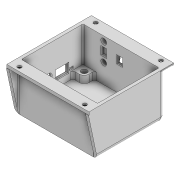
# Autodesk Inventor part: Temp
Saved by Autodesk Inventor 2021.2 (Build 252289000, 289)
## iProperties
Created: 2023-12-02
Part Number: Temp
Material: Типовые
Document SubType Name: Modeling
Designer: Egor
Density: 1 g/cm^3
Appearance: По умолчанию
Author: Egor
Autodesk Inventor part; units mm, degrees
ref_plane "YZ Plane" through (0, 0, 0) normal (1, 0, 0) x (0, 1, 0)
ref_plane "XZ Plane" through (0, 0, 0) normal (0, 1, 0) x (-1, 0, 0)
ref_plane "XY Plane" through (0, 0, 0) normal (0, 0, 1) x (1, 0, 0)
sketch "Эскиз1" plane through (0, 0, 0) normal (0, 1, 0) x (-1, 0, 0)
  line L0 (0, -50) -> (58, -50)
  line L1 (-2, -2) -> (-2, -48)
  line L2 (58, 0) -> (0, 0)
  line L3 (60, -48) -> (60, -2)
  line L4 (-2, 0) -> (60, 0)
  line L5 (60, 0) -> (60, -50)
  line L6 (60, -50) -> (-2, -50)
  line L7 (-2, -50) -> (-2, 0)
  circle A0 centre (2, -4) radius 1.6
  circle A1 centre (55, -4) radius 1.6
  circle A2 centre (55, -46) radius 1.6
  circle A3 centre (2, -46) radius 1.6
  circle A4 centre (2, -4) radius 1.6
  circle A5 centre (55, -4) radius 1.6
  circle A6 centre (55, -46) radius 1.6
  circle A7 centre (2, -46) radius 1.6
  circle A8 centre (2, -4) radius 2.4
  circle A9 centre (2, -4) radius 4
  circle A10 centre (55, -4) radius 4
  circle A11 centre (55, -4) radius 2.4
  circle A12 centre (55, -46) radius 4
  circle A13 centre (55, -46) radius 2.4
  circle A14 centre (2, -46) radius 4
  circle A15 centre (2, -46) radius 2.4
  dimension "d0" = 4.8
  dimension "d1" = 8
  dimension "d2" = 4.8
  dimension "d3" = 8
  dimension "d4" = 4.8
  dimension "d5" = 8
  dimension "d6" = 4.8
  dimension "d7" = 8
  constraints: 16 centre point, 16 end point, 9 coincident, 4 concentric, 2 parallel, 1 horizontal, 1 perpendicular, 1 point on line
  measures "d0" diameter of A8
  measures "d1" diameter of A9
  measures "d2" diameter of A11
  measures "d3" diameter of A10
  measures "d4" diameter of A13
  measures "d5" diameter of A12
  measures "d6" diameter of A15
  measures "d7" diameter of A14
extrude "Выдавливание1" add sketch "Эскиз1" along normal blind 2.5 contours L6 L7 L1 A14 L0 | A12 | A10 | A14 L1 A9 L2 L4 L5 L3 L6 L0 | A14 | L1 L7 L4 L2 A9 | A9 | A0 | A1 | A2 | A3 | A8 | A11 | A13 | A15
extrude "Выдавливание2" add sketch "Эскиз1" along normal blind 8.5 contours A12 | A10 | A14 | A9
sketch "Эскиз2" plane through (0, 0, 0) normal (0, -1, 0) x (1, 0, 0)
  line L0 (-60, 0) -> (2, 0) projected
  line L1 (2, 0) -> (2, -50) projected
  line L2 (2, -50) -> (-60, -50) projected
  line L3 (-60, -50) -> (-60, 0) projected
  line L4 (2, 0) -> (2, -50) projected
  line L5 (2.5, -50.5) -> (-60.5, -50.5)
  line L6 (-60.5, -50.5) -> (-60.5, 0.5)
  line L7 (-60.5, 0.5) -> (2.5, 0.5)
  line L8 (2.5, 0.5) -> (2.5, -50.5)
  line L9 (5, -50.5) -> (5, -53)
  line L10 (5, -53) -> (2.5, -53)
  line L11 (5, -53) -> (-63, -53)
  line L12 (-63, -53) -> (-63, 3)
  line L13 (-63, 3) -> (5, 3)
  line L14 (5, 3) -> (5, -53)
  point P0 (0, 0)
  dimension "d14" = 63
  dimension "d15" = 51
  dimension "d16" = 2.5
  dimension "d17" = 2.5
  dimension "d18" = 68
  dimension "d19" = 56
  constraints: 20 end point, 4 parallel, 2 horizontal, 2 perpendicular
  measures "d14" distance of L6.end L7.end
  measures "d15" distance of L5.end L6.end
  measures "d16" distance of L9.end L10.end
  measures "d17" distance of L9.start L9.end
  measures "d18" distance of L12.end L13.end
  measures "d19" distance of L11.end L12.end
extrude "Выдавливание3" add sketch "Эскиз2" against normal blind 2.5 contours L5 L6 L7 L8
extrude "Выдавливание4" add sketch "Эскиз2" against normal blind 35 contours L9 L10 L11 L12 L13 L14
sketch "Эскиз3" plane through (-63, 0, 3) normal (0, 0, 1) x (1, 0, 0)
  line L0 (0, 0) -> (0, 35) projected
  line L1 (0, 35) -> (68, 35)
  line L2 (68, 35) -> (68, 50)
  line L3 (68, 50) -> (0, 50)
  line L4 (0, 50) -> (0, 35)
  point P0 (63, 0)
  dimension "d24" = 15
  constraints: 8 end point, 2 parallel, 1 horizontal, 1 perpendicular
  measures "d24" distance of L2.end L1.end
extrude "Выдавливание5" add sketch "Эскиз3" against normal blind 150
sketch "Эскиз4" plane through (-63, 50, 3) normal (0, 1, 0) x (1, 0, 0)
  line L0 (0, 0) -> (0, 56) projected
  line L1 (68, 0) -> (68, 150) projected
  line L2 (0, 0) -> (68, 0)
  line L3 (68, 0) -> (68, 150)
  line L4 (68, 150) -> (0, 150)
  line L5 (0, 150) -> (0, 0)
  point P0 (63, 3)
  constraints: 8 end point, 2 parallel, 1 horizontal, 1 perpendicular
extrude "Выдавливание6" cut sketch "Эскиз4" against normal blind 2.5
sketch "Эскиз5" plane through (-63, 47.5, 3) normal (0, 1, 0) x (1, 0, 0)
  line L0 (0, 56) -> (0, 150) projected
  line L1 (0, 150) -> (10, 150)
  line L2 (10, 150) -> (10, 140)
  line L3 (10, 140) -> (0, 140)
  line L4 (0, 140) -> (0, 150)
  line L5 (68, 150) -> (0, 150) projected
  line L6 (68, 150) -> (58, 150)
  line L7 (58, 150) -> (58, 140)
  line L8 (58, 140) -> (68, 140)
  line L9 (68, 140) -> (68, 150)
  line L10 (0, 0) -> (0, 56) projected
  line L11 (0, 0) -> (10, 0)
  line L12 (10, 0) -> (10, 10)
  line L13 (10, 10) -> (0, 10)
  line L14 (0, 10) -> (0, 0)
  line L15 (10, 10) -> (58, 10)
  line L16 (58, 10) -> (58, 140)
  line L17 (58, 140) -> (10, 140)
  line L18 (10, 140) -> (10, 10)
  point P0 (63, 3)
  dimension "d29" = 10
  dimension "d30" = 10
  dimension "d31" = 10
  dimension "d32" = 10
  dimension "d33" = 10
  dimension "d34" = 10
  constraints: 32 end point, 8 parallel, 4 horizontal, 4 perpendicular
  measures "d29" distance of L2.end L3.end
  measures "d30" distance of L1.end L2.end
  measures "d31" distance of L8.end L7.end
  measures "d32" distance of L7.end L6.end
  measures "d33" distance of L13.end L12.end
  measures "d34" distance of L12.end L11.end
extrude "Выдавливание7" cut sketch "Эскиз5" against normal blind 10 contours L17 L16 L15 L18
sketch "Эскиз6" plane through (-63, 37.5, 3) normal (0, 1, 0) x (1, 0, 0)
  line L0 (58, 140) -> (10, 140) projected
  line L1 (10, 140) -> (10, 10) projected
  line L2 (10, 10) -> (58, 10) projected
  line L3 (58, 10) -> (58, 140) projected
  line L4 (0, 150) -> (68, 150) projected
  line L5 (68, 150) -> (68, 0) projected
  line L6 (68, 0) -> (0, 0) projected
  line L7 (0, 0) -> (0, 150) projected
  line L8 (68, 56) -> (0, 56) projected
  line L9 (0, 56) -> (10, 56)
  line L10 (10, 56) -> (10, 46)
  line L11 (10, 46) -> (0, 46)
  line L12 (0, 46) -> (0, 56)
  line L13 (10, 46) -> (58, 46)
  line L14 (58, 46) -> (58, 10)
  line L15 (58, 10) -> (10, 10)
  line L16 (10, 10) -> (10, 46)
  point P0 (63, 3)
  dimension "d37" = 10
  dimension "d38" = 10
  constraints: 16 end point, 4 parallel, 2 horizontal, 2 perpendicular
  measures "d37" distance of L10.end L11.end
  measures "d38" distance of L9.end L10.end
extrude "Выдавливание8" cut sketch "Эскиз6" against normal blind 10 contours L3 L2 L1 L13
sketch "Эскиз7" plane through (-63, 47.5, 3) normal (0, 1, 0) x (1, 0, 0)
  line L0 (0, 0) -> (0, 150) projected
  line L1 (0, 150) -> (2.5, 150)
  line L2 (2.5, 150) -> (2.5, 147.5)
  line L3 (2.5, 147.5) -> (0, 147.5)
  line L4 (0, 147.5) -> (0, 150)
  line L5 (68, 150) -> (68, 0) projected
  line L6 (68, 150) -> (65.5, 150)
  line L7 (65.5, 150) -> (65.5, 147.5)
  line L8 (65.5, 147.5) -> (68, 147.5)
  line L9 (68, 147.5) -> (68, 150)
  line L10 (2.5, 2.5) -> (2.5, 53.5) projected
  line L11 (65.5, 147.5) -> (2.5, 147.5)
  line L12 (2.5, 147.5) -> (2.5, 10)
  line L13 (2.5, 10) -> (65.5, 10)
  line L14 (65.5, 10) -> (65.5, 147.5)
  point P0 (63, 3)
  dimension "d41" = 2.5
  dimension "d42" = 2.5
  dimension "d43" = 2.5
  dimension "d44" = 2.5
  dimension "d45" = 137.5
  constraints: 24 end point, 6 parallel, 3 horizontal, 3 perpendicular, 1 point on line
  measures "d41" distance of L2.end L3.end
  measures "d42" distance of L1.end L2.end
  measures "d43" distance of L8.end L7.end
  measures "d44" distance of L7.end L6.end
  measures "d45" distance of L12.end L11.end
extrude "Выдавливание9" cut sketch "Эскиз7" against normal blind 10 contours L11 L14 L13 L10 L12
sketch "Эскиз8" plane through (-63, 37.5, 3) normal (0, 1, 0) x (1, 0, 0)
  line L0 (58, 10) -> (58, 46) projected
  line L1 (58, 46) -> (10, 46) projected
  line L2 (10, 46) -> (10, 10) projected
  line L3 (2.5, 10) -> (10, 10) projected
  line L4 (2.5, 147.5) -> (2.5, 10) projected
  line L5 (65.5, 147.5) -> (2.5, 147.5) projected
  line L6 (65.5, 10) -> (65.5, 147.5) projected
  line L7 (58, 10) -> (65.5, 10) projected
  line L8 (10, 10) -> (58, 10) projected
  line L9 (0, 150) -> (68, 150) projected
  line L10 (68, 150) -> (68, 0) projected
  line L11 (68, 0) -> (0, 0) projected
  line L12 (0, 0) -> (0, 150) projected
  circle A0 centre (8, 49) radius 2.4 projected
  line L13 (2.5, 53.5) -> (65.5, 53.5) projected
  line L14 (65.5, 147.5) -> (65.5, 10) projected
  circle A1 centre (61, 49) radius 4 projected
  circle A2 centre (8, 7) radius 4 projected
  circle A3 centre (8, 49) radius 4 projected
  line L15 (2.5, 2.5) -> (65.5, 2.5) projected
  line L16 (65.5, 2.5) -> (65.5, 53.5) projected
  line L17 (65.5, 53.5) -> (2.5, 53.5) projected
  line L18 (2.5, 53.5) -> (2.5, 2.5) projected
  circle A4 centre (61, 7) radius 4 projected
  circle A5 centre (8, 7) radius 4 projected
  line L19 (2.5, 2.5) -> (2.5, 53.5) projected
  line L20 (65.5, 2.5) -> (2.5, 2.5) projected
  line L21 (65.5, 53.5) -> (65.5, 2.5) projected
  circle A6 centre (61, 7) radius 2.4 projected
  line L22 (2.5, 53.5) -> (65.5, 53.5)
  line L23 (65.5, 53.5) -> (65.5, 2.5)
  line L24 (65.5, 2.5) -> (2.5, 2.5)
  line L25 (2.5, 2.5) -> (2.5, 53.5)
  point P0 (63, 3)
  point P1 (58.3542, 10)
  point P2 (63.6458, 10)
  point P3 (10.6458, 10)
  point P4 (10, 10.4641)
  point P5 (10, 45.5359)
  point P6 (10.6458, 46)
  constraints: 8 end point, 2 parallel, 1 horizontal, 1 perpendicular
extrude "Выдавливание10" cut sketch "Эскиз8" along normal mid plane 20 contours L0 L1 A3 L2 A2 L3 L4 L13 L6 L7 A4 | L7 A4 L16 L15 L18 L3 A2 L8 | A4 L7 | L7 A4 | A2 L3 L8 | L8 L2 A2 | A3 L2 L1 | L1 L2 A3 | L3 A2 L2 | A0 | A1 | A6
sketch "Эскиз9" plane through (-63, 0, 3) normal (0, 0, 1) x (1, 0, 0)
  line L0 (68, 0) -> (68, 47.5) projected
  line L1 (68, 35) -> (0, 35) projected
  line L2 (68, 47.5) -> (0, 47.5)
  line L3 (0, 47.5) -> (0, 35)
  line L4 (0, 35) -> (68, 35)
  line L5 (68, 35) -> (68, 47.5)
  point P0 (63, 0)
  constraints: 8 end point, 2 parallel, 1 horizontal, 1 perpendicular
extrude "Выдавливание11" add sketch "Эскиз9" along normal blind 10
sketch "Эскиз12" plane through (-63, 37.5, 3) normal (0, 1, 0) x (1, 0, 0)
  line L0 (65.5, 2.5) -> (65.5, 53.5) projected
  line L1 (65.5, 53.5) -> (55.5, 53.5)
  line L2 (55.5, 53.5) -> (55.5, 63.5)
  line L3 (55.5, 63.5) -> (65.5, 63.5)
  line L4 (65.5, 63.5) -> (65.5, 53.5)
  line L5 (2.5, 53.5) -> (2.5, 2.5) projected
  line L6 (2.5, 53.5) -> (12.5, 53.5)
  line L7 (12.5, 53.5) -> (12.5, 63.5)
  line L8 (12.5, 63.5) -> (2.5, 63.5)
  line L9 (2.5, 63.5) -> (2.5, 53.5)
  point P0 (63, 3)
  dimension "d52" = 10
  dimension "d53" = 10
  dimension "d54" = 10
  constraints: 16 end point, 4 parallel, 2 horizontal, 2 perpendicular
  measures "d52" distance of L2.end L3.end
  measures "d53" distance of L1.end L2.end
  measures "d54" distance of L8.end L7.end
extrude "Выдавливание12" add sketch "Эскиз12" along normal blind 10
sketch "Эскиз14" plane through (-63, 47.5, 3) normal (0, 1, 0) x (1, 0, 0)
  line L0 (-39.8983, 166.515) -> (151.9505, 166.515)
  line L1 (151.9505, 166.515) -> (151.9505, -49.8726)
  line L2 (151.9505, -49.8726) -> (-39.8983, -49.8726)
  line L3 (-39.8983, -49.8726) -> (-39.8983, 166.515)
  point P0 (63, 3)
  constraints: 8 end point, 2 parallel, 1 horizontal, 1 perpendicular
extrude "Выдавливание13" cut sketch "Эскиз14" against normal blind 10
sketch "Эскиз15" plane through (0, 0, 0) normal (0, -1, 0) x (1, 0, 0)
  line L0 (5, -53) -> (5, 3) projected
  line L1 (5, -53) -> (-63, -53) projected
  line L2 (5, 3) -> (-63, 3)
  line L3 (-63, 3) -> (-63, -53)
  line L4 (-63, -53) -> (5, -53)
  line L5 (5, -53) -> (5, 3)
  line L6 (5, 3) -> (5, 13) projected
  line L7 (-63, 3) -> (-63, 13) projected
  line L8 (5, 3) -> (-63, 3)
  line L9 (-63, 3) -> (-63, 13)
  line L10 (-63, 13) -> (5, 13)
  line L11 (5, 13) -> (5, 3)
  line L12 (5, 3) -> (-63, 3) projected
  line L13 (5, 3) -> (-63, 3)
  line L14 (-63, 3) -> (-63, 10)
  line L15 (-63, 10) -> (5, 10)
  line L16 (5, 10) -> (5, 3)
  line L17 (-63, 13) -> (-63, -147) projected
  line L18 (5, -53) -> (-63, -53)
  line L19 (-63, -53) -> (-63, -60)
  line L20 (-63, -60) -> (5, -60)
  line L21 (5, -60) -> (5, -53)
  line L22 (5, -60) -> (-63, -60)
  line L23 (-63, -60) -> (-63, -147)
  line L24 (-63, -147) -> (5, -147)
  line L25 (5, -147) -> (5, -60)
  point P0 (0, 0)
  point P1 (5, 10)
  dimension "d59" = 7
  dimension "d60" = 7
  constraints: 40 end point, 10 parallel, 5 horizontal, 5 perpendicular, 2 point on line
  measures "d59" distance of L13.end L14.end
  measures "d60" distance of L19.end L18.end
extrude "Выдавливание14" cut sketch "Эскиз15" against normal blind 100 contours L25 L24 L17 L20 | L15 L7 L10 L6
sketch "Эскиз16" plane through (-63, 35, -53) normal (0, -1, 0) x (1, 0, 0)
  line L0 (0, 0) -> (68, 0) projected
  line L1 (0, -7) -> (68, -7) projected
  line L2 (68, -7) -> (0, -7) projected
  line L3 (0, -7) -> (0, 0) projected
  line L4 (0, 0) -> (0, 56) projected
  line L5 (0, 56) -> (0, 63) projected
  line L6 (0, 63) -> (68, 63) projected
  line L7 (68, 63) -> (68, 56) projected
  line L8 (68, 56) -> (68, 0) projected
  line L9 (68, 0) -> (68, -7) projected
  line L10 (68, 0) -> (0, 0) projected
  line L11 (0, 56) -> (68, 56) projected
  line L12 (2.5, 53.5) -> (2.5, 2.5) projected
  line L13 (2.5, 2.5) -> (65.5, 2.5) projected
  line L14 (65.5, 2.5) -> (65.5, 53.5) projected
  line L15 (65.5, 53.5) -> (2.5, 53.5) projected
  line L16 (68, -7) -> (0, -7) projected
  line L17 (0, -7) -> (0, 0) projected
  line L18 (0, 0) -> (0, 56) projected
  line L19 (0, 56) -> (0, 63) projected
  line L20 (0, 63) -> (68, 63) projected
  line L21 (68, 63) -> (68, 56) projected
  line L22 (68, 56) -> (68, 0) projected
  line L23 (68, 0) -> (68, -7) projected
  line L24 (68, 0) -> (0, 0) projected
  line L25 (0, 56) -> (68, 56) projected
  line L26 (2.5, 53.5) -> (2.5, 2.5) projected
  line L27 (2.5, 2.5) -> (65.5, 2.5) projected
  line L28 (65.5, 2.5) -> (65.5, 53.5) projected
  line L29 (65.5, 53.5) -> (2.5, 53.5) projected
  line L30 (68, -7) -> (0, -7) projected
  line L31 (0, -7) -> (0, 0) projected
  line L32 (0, 0) -> (0, 56) projected
  line L33 (0, 56) -> (0, 63) projected
  line L34 (0, 63) -> (68, 63) projected
  line L35 (68, 63) -> (68, 56) projected
  line L36 (68, 56) -> (68, 0) projected
  line L37 (68, 0) -> (68, -7) projected
  line L38 (68, 0) -> (0, 0) projected
  line L39 (0, 56) -> (68, 56) projected
  line L40 (2.5, 53.5) -> (2.5, 2.5) projected
  line L41 (2.5, 2.5) -> (65.5, 2.5) projected
  line L42 (65.5, 2.5) -> (65.5, 53.5) projected
  line L43 (65.5, 53.5) -> (2.5, 53.5) projected
  line L44 (68, 0) -> (68, -7) projected
  line L45 (68, 0) -> (0, 0) projected
  line L46 (68, -7) -> (61, -7)
  line L47 (61, -7) -> (61, 0)
  line L48 (61, 0) -> (68, 0)
  line L49 (68, 0) -> (68, -7)
  circle A0 centre (61, -3.5) radius 1.6
  line L50 (0, 0) -> (0, -7) projected
  line L51 (0, -7) -> (7, -7)
  line L52 (7, -7) -> (7, 0)
  line L53 (7, 0) -> (0, 0)
  line L54 (0, 0) -> (0, -7)
  circle A1 centre (7, -3.5) radius 1.6
  line L55 (68, -7) -> (68, 63) projected
  line L56 (68, 56) -> (0, 56) projected
  line L57 (68, 63) -> (61, 63)
  line L58 (61, 63) -> (61, 56)
  line L59 (61, 56) -> (68, 56)
  line L60 (68, 56) -> (68, 63)
  line L61 (0, 56) -> (0, 63) projected
  line L62 (0, 63) -> (7, 63)
  line L63 (7, 63) -> (7, 56)
  line L64 (7, 56) -> (0, 56)
  line L65 (0, 56) -> (0, 63)
  circle A2 centre (61, 59.5) radius 1.6
  circle A3 centre (7, 59.5) radius 1.6
  point P0 (63, 53)
  dimension "d63" = 7
  dimension "d64" = 3.2
  dimension "d65" = 7
  dimension "d66" = 7
  constraints: 32 end point, 8 parallel, 4 centre point, 4 horizontal, 4 midpoint, 4 perpendicular, 4 point on line
  measures "d63" distance of L47.end L48.end
  measures "d64" diameter of A0
  measures "d65" distance of L53.end L52.end
  measures "d66" distance of L59.end L58.end
extrude "Выдавливание15" cut sketch "Эскиз16" against normal blind 100 contours A1 L52 | L52 A1 | A0 L47 | L47 A0 | A3 L63 | L63 A3 | A2 L58 | L58 A2
chamfer "Фаска1" distance 1.2 angle 45 4 edges at (-3.6, 35, -56.5) (-57.6, 35, -56.5) (-3.6, 35, 6.5) (-57.6, 35, 6.5)
sketch "Эскиз17" plane through (5, 0, 3) normal (1, 0, 0) x (0, 0, -1)
  line L0 (-7, 37.5) -> (-7, 35) projected
  line L1 (-7, 37.5) -> (-10, 37.5)
  line L2 (-7, 35) -> (-10, 35)
  line L3 (0, 0) -> (0, 35) projected
  line L4 (-10, 35) -> (0, 0)
  line L5 (0, 0) -> (0, 35)
  line L6 (0, 35) -> (-11.0943, 35)
  point P0 (3, 0)
  dimension "d72" = 3
  constraints: 10 end point, 2 horizontal, 2 point on line, 1 perpendicular
  measures "d72" distance of L0.start L1.end
extrude "Выдавливание16" add sketch "Эскиз17" against normal blind 2.5
sketch "Эскиз18" plane through (-63, 0, -53) normal (-1, 0, 0) x (0, 0, 1)
  line L0 (56, 0) -> (66, 35) projected
  line L1 (66, 35) -> (63, 35) projected
  line L2 (56, 35) -> (63, 35) projected
  line L3 (56, 0) -> (56, 35) projected
  line L4 (56, 0) -> (66, 35) projected
  line L5 (0, 0) -> (56, 0) projected
  line L6 (63, 35) -> (66, 35) projected
  line L7 (56, 0) -> (66, 35)
  line L8 (66, 35) -> (56, 35)
  line L9 (56.7, 35) -> (62.3, 35) projected
  line L10 (56, 0) -> (56, 35) projected
  line L11 (56, 0) -> (56, 35)
  point P0 (53, 0)
  constraints: 6 end point, 2 collinear
extrude "Выдавливание17" add sketch "Эскиз18" against normal blind 2.5
sketch "Эскиз19" plane through (5, 0, -53) normal (1, 0, 0) x (0, 0, -1)
  line L0 (-66, 35) -> (-66, 47.5)
  line L1 (-56, 0) -> (-66, 35)
  line L2 (-56, 0) -> (-66, 47.5)
  line L3 (-66, 35) -> (-56, 0)
  line L4 (-66, 47.5) -> (-66, 35)
  line L5 (-66, 35) -> (-56, 0) projected
  line L6 (0, 0) -> (-56, 0) projected
  point P0 (-53, 0)
  point P1 (-55.5522, -2.2285)
  constraints: 10 end point
extrude "Выдавливание18" cut sketch "Эскиз19" against normal through all
fillet "Сопряжение1" radius 2 2 edges at (5, 35, -56.5) (-63, 35, -56.5)
fillet "Сопряжение2" radius 4 7 edges at (5, 0, -25) (-29, 0, -53) (-63, 0, -25) (-63, 36, -53) (-63, 17.5, -53) (5, 36, -53) (5, 17.5, -53)
sketch "Эскиз20" plane through (-63, 37.5, -60) normal (-1, 0, 0) x (0, 0, 1)
  line L0 (58, -29) -> (12, -29)
  circle A0 centre (37.9, -24.1936) radius 0.9504
  circle A1 centre (37.9, -24.1936) radius 1.3947
  line L1 (39.17, -22.1571) -> (36.63, -22.1571)
  arc A2 (36.63, -22.1571) -> (36.63, -26.23) centre (37.9, -24.1936) ccw
  arc A3 (39.17, -26.23) -> (39.17, -22.1571) centre (37.9, -24.1936) ccw
  circle A4 centre (37.9, -24.1936) radius 2.45
  circle A5 centre (47.525, -23.4086) radius 1.3526
  circle A6 centre (47.525, -23.4086) radius 1.5525
  circle A7 centre (47.525, -23.4086) radius 1.7
  line L2 (23.65, -23.7586) -> (29.95, -23.7586)
  line L3 (26.8, -23.7586) -> (26.8, -29)
  line L4 (26.8, -29) -> (21.8, -29)
  line L5 (26.8, -29) -> (31.8, -29)
  line L6 (31.8, -29) -> (31.8, -22)
  line L7 (31.8, -22) -> (21.8, -22)
  line L8 (21.8, -22) -> (21.8, -29)
  point P0 (60, -37.5)
  point P1 (36.63, -26.23)
  point P2 (36.63, -22.1571)
  dimension "d81" = 4.9
  dimension "d82" = 3.4
  dimension "d83" = 5
  dimension "d84" = 5
  dimension "d85" = 7
  constraints: 18 end point, 8 centre point, 4 perpendicular, 4 point on circle, 3 point on line, 2 coincident, 1 midpoint
  measures "d81" diameter of A4
  measures "d82" diameter of A7
  measures "d83" distance of L3.end L8.end
  measures "d84" distance of L3.end L6.start
  measures "d85" distance of L6.start L6.end
extrude "Выдавливание19" cut sketch "Эскиз20" against normal blind 10 contours L0 L8 L7 L6 | A0 | A1 | A4 | A5 | A6 | A7
sketch "Эскиз21" plane through (0, 2.5, 0) normal (0, 1, 0) x (1, 0, 0)
  line L0 (-60.5, 50.5) -> (2.5, 50.5) projected
  line L1 (-60.5, 50.5) -> (-60.5, -0.5) projected
  circle A0 centre (-2, 46) radius 4 projected
  circle A1 centre (-55, 4) radius 4 projected
  circle A2 centre (-55, 46) radius 4 projected
  line L2 (-60.5, -0.5) -> (2.5, -0.5) projected
  line L3 (2.5, -0.5) -> (2.5, 50.5) projected
  line L4 (2.5, 50.5) -> (-60.5, 50.5) projected
  line L5 (-60.5, 50.5) -> (-60.5, -0.5) projected
  circle A3 centre (-2, 4) radius 4 projected
  circle A4 centre (-55, 46) radius 4 projected
  circle A5 centre (-2, 46) radius 4 projected
  circle A6 centre (-2, 4) radius 4 projected
  circle A7 centre (-55, 4) radius 4 projected
  line L6 (-60.5, -0.5) -> (2.5, -0.5) projected
  line L7 (-60.5, 50.5) -> (-55, 50.5)
  line L8 (-60.5, 50.5) -> (-60.5, 46)
  line L9 (-60.5, 50.5) -> (-60.5, -0.5) projected
  line L10 (-55, 42) -> (-60.5, 42)
  line L11 (-60.5, 46) -> (-60.5, 42)
  line L12 (-51, 46) -> (-51, 50.5)
  line L13 (-51, 50.5) -> (-60.5, 50.5)
  line L14 (-6, 46) -> (-6, 50.5)
  line L15 (-6, 50.5) -> (2.5, 50.5)
  line L16 (2.5, 50.5) -> (2.5, 42)
  line L17 (2.5, -0.5) -> (2.5, 50.5) projected
  line L18 (-2, 42) -> (2.5, 42)
  circle A8 centre (-55, 4) radius 4 projected
  line L19 (-55, 8) -> (-60.5, 8)
  line L20 (-60.5, 8) -> (-60.5, -0.5)
  line L21 (-60.5, -0.5) -> (-55, -0.5)
  line L22 (-60.5, -0.5) -> (2.5, -0.5) projected
  line L23 (-51, 4) -> (-51, -0.5)
  line L24 (-51, -0.5) -> (-60.5, -0.5)
  circle A9 centre (-2, 4) radius 4 projected
  line L25 (-6, 4) -> (-6, -0.5)
  line L26 (-2, 8) -> (2.5, 8)
  line L27 (2.5, 8) -> (2.5, -0.5)
  line L28 (2.5, -0.5) -> (-6, -0.5)
  point P0 (0, 0)
  point P1 (2.5, 50.5)
  constraints: 38 end point, 13 tangent, 11 point on line, 9 perpendicular, 7 collinear, 6 point on circle, 1 horizontal, 1 horizontal alignment, 1 vertical, 1 vertical alignment, 2 other
extrude "Выдавливание20" add sketch "Эскиз21" along normal up to surface (6 mm away) contours L0 L12 A2 L10 L1 | L0 L3 L18 A0 L14 | L19 A1 L23 L2 L1 | L3 L2 L25 A3 L26
fillet "Сопряжение3" radius 2 8 edges at (-60.5, 5.5, -42) (-51, 5.5, -50.5) (-6, 5.5, -50.5) (2.5, 5.5, -42) (2.5, 5.5, -8) (-6, 5.5, 0.5) (-51, 5.5, 0.5) (-60.5, 5.5, -8)
fillet "Сопряжение4" radius 1 6 edges at (-60.5, 23, -50.5) (2.5, 23, -50.5) (2.5, 23, 0.5) (-60.5, 23, 0.5) (2.5, 17.646, 3) (-60.5, 17.646, 3)
fillet "Сопряжение5" radius 0.5 8 edges at (-63, 8.5, -33.2) (-63, 12, -38.2) (-63, 12, -28.2) (-63, 15.5, -33.2) (-60.5, 8.5, -33.2) (-60.5, 12, -28.2) (-60.5, 15.5, -33.2) (-60.5, 12, -38.2)
fillet "Сопряжение6" radius 0.5 2 edges at (-63, 13.3064, -24.55) (-63, 14.0914, -14.175)
fillet "Сопряжение7" radius 0.5 2 edges at (-60.5, 13.3064, -24.55) (-60.5, 14.0914, -14.175)
sketch "Эскиз22" plane through (-63, 37.5, -60) normal (-1, 0, 0) x (0, 0, 1)
  line L0 (7, -2.5) -> (7, -33.5)
  line L1 (18, -27.4086) -> (20, -27.4086)
  line L2 (20, -27.4086) -> (20, -26.4086)
  line L3 (20, -26.4086) -> (18, -26.4086)
  line L4 (18, -26.4086) -> (18, -27.4086)
  point P0 (60, -37.5)
  point P1 (12, -27.4086)
  dimension "d96" = 2
  dimension "d97" = 1
  constraints: 10 end point, 2 perpendicular
  measures "d96" distance of L1.start L1.end
  measures "d97" distance of L1.end L2.end
extrude "Выдавливание21" cut sketch "Эскиз22" against normal blind 10
fillet "Сопряжение8" radius 0.5 8 edges at (-60.5, 10.0914, -41) (-60.5, 11.0914, -41) (-60.5, 10.5914, -42) (-60.5, 10.5914, -40) (-63, 10.5914, -42) (-63, 11.0914, -41) (-63, 10.0914, -41) (-63, 10.5914, -40)
sketch "Эскиз23" plane through (1, 35, -53) normal (0, 0, -1) x (-1, 0, 0)
  line L0 (33.3181, -5.842) -> (29.3181, -5.842)
  line L1 (29.3181, -11.842) -> (33.3181, -11.842)
  line L2 (29.3181, -5.842) -> (29.3181, -11.842)
  line L3 (33.3181, -11.842) -> (33.3181, -5.842)
  line L4 (62, 0) -> (-2, 0)
  line L5 (60, 0) -> (60, -31)
  line L6 (61.5, 2.5) -> (61.5, -26.5)
  line L7 (33.3181, 0) -> (33.3181, -6)
  line L8 (33.3181, -6) -> (29.3181, -6)
  line L9 (29.3181, -6) -> (29.3181, -12)
  line L10 (29.3181, -12) -> (33.3181, -12)
  line L11 (33.3181, -12) -> (33.3181, -6)
  point P0 (1, -35)
  dimension "d101" = 6
  dimension "d102" = 4
  dimension "d103" = 6
  constraints: 24 end point, 2 parallel, 2 point on line, 1 horizontal, 1 perpendicular
  measures "d101" distance of L7.start L7.end
  measures "d102" distance of L10.end L9.end
  measures "d103" distance of L9.end L8.end
extrude "Выдавливание22" cut sketch "Эскиз23" against normal blind 10 contours L3 L1 L2 L8
fillet "Сопряжение9" radius 0.5 8 edges at (-28.3181, 26.079, -53) (-30.3181, 29, -53) (-30.3181, 23.158, -53) (-32.3181, 26.079, -53) (-30.3181, 23.158, -50.5) (-28.3181, 26.079, -50.5) (-30.3181, 29, -50.5) (-32.3181, 26.079, -50.5)
sketch "Эскиз24" plane through (1, 35, -53) normal (0, 0, -1) x (-1, 0, 0)
  line L0 (29.3181, -6) -> (33.3181, -6)
  line L1 (29.3181, -11.842) -> (29.3181, -6)
  line L2 (33.3181, -6) -> (33.3181, -11.842)
  line L3 (33.3181, -11.842) -> (29.3181, -11.842)
  line L4 (33.3181, -6) -> (44.3181, -6)
  line L5 (33.3181, -6) -> (33.3181, -1.5)
  line L6 (33.3181, -1.5) -> (44.3181, -1.5)
  circle A0 centre (44.3181, -1.5) radius 1.5
  line L7 (44.3181, -1.5) -> (44.3181, -16.5)
  circle A1 centre (44.3181, -16.5) radius 1.5
  circle A2 centre (44.3181, -1.5) radius 2.4
  circle A3 centre (44.3181, -16.5) radius 4
  circle A4 centre (44.3181, -1.5) radius 4
  circle A5 centre (44.3181, -16.5) radius 2.4
  point P0 (1, -35)
  dimension "d107" = 11
  dimension "d108" = 4.5
  dimension "d109" = 3
  dimension "d110" = 15
  dimension "d111" = 3
  dimension "d112" = 4.8
  dimension "d113" = 8
  dimension "d114" = 8
  dimension "d115" = 4.8
  constraints: 16 end point, 6 centre point, 6 coincident, 2 vertical, 1 horizontal, 1 perpendicular
  measures "d107" distance of L5.start L4.end
  measures "d108" distance of L5.start L6.start
  measures "d109" diameter of A0
  measures "d110" distance of L7.start L7.end
  measures "d111" diameter of A1
  measures "d112" diameter of A2
  measures "d113" diameter of A3
  measures "d114" diameter of A4
  measures "d115" diameter of A5
extrude "Выдавливание23" cut sketch "Эскиз24" against normal blind 10 contours L7 L6 A0 | A0 L6 L7 | A1
sketch "Эскиз25" plane through (1, 4, -53) normal (0, 0, -1) x (-1, 0, 0)
  circle A0 centre (44.3181, 14.5) radius 1.5 projected
  circle A1 centre (44.3181, 14.5) radius 2.4
  circle A2 centre (44.3181, 29.5) radius 1.5 projected
  circle A3 centre (44.3181, 29.5) radius 2.4
  circle A4 centre (44.3181, 14.5) radius 4
  circle A5 centre (44.3181, 29.5) radius 4
  point P0 (1, -4)
  dimension "d118" = 4.8
  dimension "d119" = 4.8
  dimension "d120" = 8
  dimension "d121" = 8
  constraints: 4 centre point, 4 coincident
  measures "d118" diameter of A1
  measures "d119" diameter of A3
  measures "d120" diameter of A4
  measures "d121" diameter of A5
extrude "Выдавливание24" add sketch "Эскиз25" along normal up to surface (7 mm away) contours A4 | A5
sketch "Эскиз26" plane through (-49, 2.5, -50.5) normal (0, 0, 1) x (1, 0, 0)
  circle A0 centre (5.6819, 16) radius 1.5 projected
  circle A1 centre (5.6819, 31) radius 1.5 projected
  line L0 (21.1819, 20.158) -> (16.1819, 20.158) projected
  line L1 (16.1819, 20.158) -> (16.1819, 27) projected
  line L2 (16.1819, 27) -> (21.1819, 27) projected
  line L3 (21.1819, 27) -> (21.1819, 20.158) projected
  arc A2 (50, -2.2081) -> (53.7081, 1.5) centre (50, 1.5) ccw projected
  line L4 (50, -2.2081) -> (-10, -2.2081) projected
  arc A3 (-13.7081, 1.5) -> (-10, -2.2081) centre (-10, 1.5) ccw projected
  line L5 (-13.7081, 1.5) -> (-13.7081, 33.4596) projected
  arc A4 (-14, 34.5) -> (-13.7081, 33.4596) centre (-12, 34.5) ccw projected
  line L6 (-14, 34.5) -> (-14, 35) projected
  line L7 (-14, 35) -> (-10.5, 35) projected
  line L8 (-10.5, 35) -> (50.5, 35) projected
  line L9 (50.5, 35) -> (54, 35) projected
  line L10 (54, 35) -> (54, 34.5) projected
  arc A5 (53.7081, 33.4596) -> (54, 34.5) centre (52, 34.5) ccw projected
  line L11 (53.7081, 33.4596) -> (53.7081, 1.5) projected
  line L12 (-10.5, 35) -> (-10.5, 6) projected
  line L13 (-10.5, 6) -> (0, 6) projected
  line L14 (0, 0) -> (0, 6) projected
  line L15 (0, 0) -> (41, 0) projected
  line L16 (41, 6) -> (41, 0) projected
  line L17 (41, 6) -> (50.5, 6) projected
  line L18 (50.5, 35) -> (50.5, 6) projected
  arc A6 (3.8084, 32.5) -> (7.5554, 32.5) centre (5.6819, 31) ccw projected
  circle A7 centre (5.6819, 16) radius 2.4 projected
  line L19 (3.2819, 31) -> (8.0819, 31)
  line L20 (8.0819, 31) -> (8.0819, 16)
  line L21 (8.0819, 16) -> (3.2819, 16)
  line L22 (3.2819, 16) -> (3.2819, 31)
  line L23 (3.2819, 31) -> (3.2819, 27)
  line L24 (3.2819, 27) -> (8.0819, 27)
  line L25 (3.2819, 16) -> (3.2819, 20)
  line L26 (3.2819, 20) -> (8.0819, 20)
  point P0 (49, -2.5)
  dimension "d124" = 4
  dimension "d125" = 4
  constraints: 16 end point, 4 point on line, 3 perpendicular, 2 parallel, 1 horizontal, 1 horizontal alignment, 1 point on circle, 1 other
  measures "d124" distance of L19.start L23.end
  measures "d125" distance of L21.end L25.end
extrude "Выдавливание25" cut sketch "Эскиз26" against normal blind 2.5 contours L26 L22 L24 L20
sketch "Эскиз27" plane through (1, 4, -53) normal (0, 0, -1) x (-1, 0, 0)
  arc A0 (40.61, 31) -> (48.0262, 31) centre (44.3181, 29.5) ccw projected
  circle A1 centre (44.3181, 14.5) radius 4 projected
  line L0 (40.3181, 29.5) -> (48.3181, 29.5)
  line L1 (48.3181, 29.5) -> (48.3181, 14.5)
  line L2 (48.3181, 14.5) -> (40.3181, 14.5)
  line L3 (40.3181, 14.5) -> (40.3181, 29.5)
  line L4 (62, 31) -> (48.0262, 31) projected
  line L5 (40.3181, 29.5) -> (48.3181, 29.5)
  line L6 (48.3181, 29.5) -> (48.3181, 31)
  line L7 (48.3181, 31) -> (40.3181, 31)
  line L8 (40.3181, 31) -> (40.3181, 29.5)
  circle A2 centre (44.3181, 14.5) radius 2.4 projected
  arc A3 (42.4446, 31) -> (46.1916, 31) centre (44.3181, 29.5) ccw projected
  line L9 (46.1916, 31) -> (44.3181, 31) projected
  circle A4 centre (44.3181, 29.5) radius 1.5 projected
  line L10 (44.3181, 31) -> (42.4446, 31) projected
  circle A5 centre (44.3181, 14.5) radius 1.5 projected
  line L11 (33.8181, 25.5) -> (33.8181, 18.658) projected
  line L12 (33.8181, 18.658) -> (28.8181, 18.658) projected
  line L13 (28.8181, 18.658) -> (28.8181, 25.5) projected
  line L14 (28.8181, 25.5) -> (33.8181, 25.5) projected
  line L15 (64, 33.5) -> (64, 33) projected
  arc A6 (62, 31) -> (64, 33) centre (62, 33) ccw projected
  line L16 (62, 31) -> (60, 31) projected
  line L17 (60, 31) -> (48.0262, 31) projected
  arc A7 (44.3181, 25.5) -> (48.0262, 31) centre (44.3181, 29.5) ccw projected
  line L18 (44.3181, 25.5) -> (41.9181, 25.5) projected
  line L19 (41.9181, 25.5) -> (41.9181, 18.5) projected
  line L20 (41.9181, 18.5) -> (44.3181, 18.5) projected
  circle A8 centre (44.3181, 14.5) radius 4 projected
  line L21 (44.3181, 18.5) -> (46.7181, 18.5) projected
  line L22 (46.7181, 18.5) -> (46.7181, 25.5) projected
  line L23 (46.7181, 25.5) -> (44.3181, 25.5) projected
  line L24 (-4, 33.5) -> (64, 33.5) projected
  line L25 (-4, 33) -> (-4, 33.5) projected
  arc A9 (-4, 33) -> (-2, 31) centre (-2, 33) ccw projected
  line L26 (0, 31) -> (-2, 31) projected
  line L27 (0, 0) -> (0, 31) projected
  line L28 (60, 0) -> (0, 0) projected
  line L29 (60, 0) -> (60, 31) projected
  arc A10 (40.61, 31) -> (44.3181, 25.5) centre (44.3181, 29.5) ccw projected
  line L30 (40.61, 31) -> (0, 31) projected
  point P0 (1, -4)
  constraints: 16 end point, 4 parallel, 2 horizontal, 2 perpendicular, 2 point on circle, 1 point on line, 1 vertical alignment
extrude "Выдавливание26" add sketch "Эскиз27" along normal up to surface (7 mm away) contours A0 L18 L19 L20 A1 L3 | A0 L1 A1 L21 L22 L23
sketch "Эскиз28" plane through (1, 4, -53) normal (0, 0, -1) x (-1, 0, 0)
  line L0 (46.7181, 25.5) -> (41.9181, 25.5) projected
  line L1 (41.9181, 25.5) -> (41.9181, 18.5) projected
  line L2 (41.9181, 18.5) -> (46.7181, 18.5) projected
  line L3 (46.7181, 18.5) -> (46.7181, 25.5) projected
  circle A0 centre (44.3181, 14.5) radius 2.4 projected
  arc A1 (42.4446, 31) -> (46.1916, 31) centre (44.3181, 29.5) ccw projected
  line L4 (46.1916, 31) -> (44.3181, 31) projected
  circle A2 centre (44.3181, 29.5) radius 1.5 projected
  line L5 (44.3181, 31) -> (42.4446, 31) projected
  circle A3 centre (44.3181, 14.5) radius 1.5 projected
  line L6 (33.8181, 25.5) -> (33.8181, 18.658) projected
  line L7 (33.8181, 18.658) -> (28.8181, 18.658) projected
  line L8 (28.8181, 18.658) -> (28.8181, 25.5) projected
  line L9 (28.8181, 25.5) -> (33.8181, 25.5) projected
  line L10 (64, 33.5) -> (64, 33) projected
  arc A4 (62, 31) -> (64, 33) centre (62, 33) ccw projected
  line L11 (62, 31) -> (60, 31) projected
  line L12 (60, 31) -> (48.0262, 31) projected
  arc A5 (48.3181, 29.5) -> (48.0262, 31) centre (44.3181, 29.5) ccw projected
  line L13 (48.3181, 29.5) -> (48.3181, 14.5) projected
  arc A6 (40.3181, 14.5) -> (48.3181, 14.5) centre (44.3181, 14.5) ccw projected
  line L14 (40.3181, 14.5) -> (40.3181, 29.5) projected
  arc A7 (40.61, 31) -> (40.3181, 29.5) centre (44.3181, 29.5) ccw projected
  line L15 (40.61, 31) -> (0, 31) projected
  line L16 (0, 31) -> (-2, 31) projected
  arc A8 (-4, 33) -> (-2, 31) centre (-2, 33) ccw projected
  line L17 (-4, 33) -> (-4, 33.5) projected
  line L18 (-4, 33.5) -> (64, 33.5) projected
  line L19 (60, 0) -> (60, 31) projected
  line L20 (60, 0) -> (0, 0) projected
  line L21 (0, 0) -> (0, 31) projected
  point P0 (1, -4)
  constraints: 1 vertical alignment
extrude "Выдавливание27" add sketch "Эскиз28" along normal up to surface (7 mm away) contours L3 L2 L1 L0
sketch "Эскиз29" plane through (-43.3181, 18.5, -53) normal (0, 0, -1) x (-1, 0, 0)
  circle A0 centre (0, 0) radius 2.4 projected
  circle A1 centre (0, 0) radius 2.4
  arc A2 (-1.8735, 16.5) -> (1.8735, 16.5) centre (0, 15) ccw projected
  circle A3 centre (0, 15) radius 2.4
  point P0 (-43.3181, -18.5)
  constraints: 2 centre point, 2 coincident
extrude "Выдавливание28" cut sketch "Эскиз29" against normal blind 2.5
sketch "Эскиз30" plane through (1, 4, -53) normal (0, 0, -1) x (-1, 0, 0)
  circle A0 centre (44.3181, 14.5) radius 2.4 projected
  circle A1 centre (44.3181, 14.5) radius 2.4
  arc A2 (42.4446, 31) -> (46.1916, 31) centre (44.3181, 29.5) ccw projected
  circle A3 centre (44.3181, 29.5) radius 2.4
  point P0 (1, -4)
  constraints: 2 centre point, 2 coincident
extrude "Выдавливание29" add sketch "Эскиз30" along normal up to surface (7 mm away)
sketch "Эскиз31" plane through (-43.3181, 33.5, -53) normal (0, 0, 1) x (1, 0, 0)
  circle A0 centre (0, 0) radius 2.4 projected
  line L0 (2.4, -11) -> (2.4, -4) projected
  line L1 (2.4, -4) -> (-2.4, -4) projected
  line L2 (-2.4, -4) -> (-2.4, -11) projected
  line L3 (-2.4, -11) -> (2.4, -11) projected
  circle A1 centre (0, -15) radius 2.4 projected
  line L4 (10.5, -4) -> (10.5, -10.842) projected
  line L5 (10.5, -10.842) -> (15.5, -10.842) projected
  line L6 (15.5, -10.842) -> (15.5, -4) projected
  line L7 (15.5, -4) -> (10.5, -4) projected
  line L8 (-19.6819, 3.5) -> (-19.6819, 4) projected
  line L9 (-19.6819, 4) -> (48.3181, 4) projected
  line L10 (48.3181, 4) -> (48.3181, 3.5) projected
  arc A2 (46.3181, 1.5) -> (48.3181, 3.5) centre (46.3181, 3.5) ccw projected
  line L11 (46.3181, 1.5) -> (44.3181, 1.5) projected
  line L12 (44.3181, 1.5) -> (3.7081, 1.5) projected
  arc A3 (4, 0) -> (3.7081, 1.5) centre (0, 0) ccw projected
  line L13 (4, 0) -> (4, -15) projected
  arc A4 (-4, -15) -> (4, -15) centre (0, -15) ccw projected
  line L14 (-4, -15) -> (-4, 0) projected
  arc A5 (-3.7081, 1.5) -> (-4, 0) centre (0, 0) ccw projected
  line L15 (-3.7081, 1.5) -> (-15.6819, 1.5) projected
  line L16 (-15.6819, 1.5) -> (-17.6819, 1.5) projected
  arc A6 (-19.6819, 3.5) -> (-17.6819, 1.5) centre (-17.6819, 3.5) ccw projected
  line L17 (44.3181, -29.5) -> (44.3181, 1.5) projected
  line L18 (-15.6819, -29.5) -> (44.3181, -29.5) projected
  line L19 (-15.6819, -29.5) -> (-15.6819, 1.5) projected
  point P0 (43.3181, -33.5)
extrude "Выдавливание30" cut sketch "Эскиз31" against normal blind 3.5 contours A0 | A1
sketch "Эскиз32" plane through (5, 37.5, -60) normal (0, 0, -1) x (-1, 0, 0)
  arc A0 (44.61, -2.5) -> (44.3181, -4) centre (48.3181, -4) ccw projected
  line L0 (44.3181, -4) -> (52.3181, -4)
  line L1 (52.3181, -4) -> (52.3181, -2.5)
  line L2 (52.3181, -2.5) -> (44.3181, -2.5)
  line L3 (44.3181, -2.5) -> (44.3181, -4)
  line L4 (68, 0) -> (68, -0.5) projected
  arc A1 (66, -2.5) -> (68, -0.5) centre (66, -0.5) ccw projected
  line L5 (66, -2.5) -> (52.0262, -2.5) projected
  arc A2 (52.3181, -4) -> (52.0262, -2.5) centre (48.3181, -4) ccw projected
  line L6 (52.3181, -4) -> (52.3181, -19) projected
  arc A3 (44.3181, -19) -> (52.3181, -19) centre (48.3181, -19) ccw projected
  line L7 (44.3181, -19) -> (44.3181, -4) projected
  arc A4 (44.61, -2.5) -> (44.3181, -4) centre (48.3181, -4) ccw projected
  line L8 (44.61, -2.5) -> (2, -2.5) projected
  arc A5 (0, -0.5) -> (2, -2.5) centre (2, -0.5) ccw projected
  line L9 (0, -0.5) -> (0, 0) projected
  line L10 (0, 0) -> (68, 0) projected
  point P0 (5, -37.5)
  constraints: 8 end point, 2 parallel, 1 horizontal, 1 perpendicular
extrude "Выдавливание31" add sketch "Эскиз32" against normal up to surface (7 mm away) contours A0 L3 L2 | L2 L1 A2
fillet "Сопряжение10" radius 2 7 edges at (-39.3181, 35, -56.5) (-47.3181, 35, -56.5) (-43.3181, 14.5, -53) (-39.3181, 26, -53) (-39.3181, 34.25, -53) (-47.3181, 26, -53) (-47.3181, 34.25, -53)
